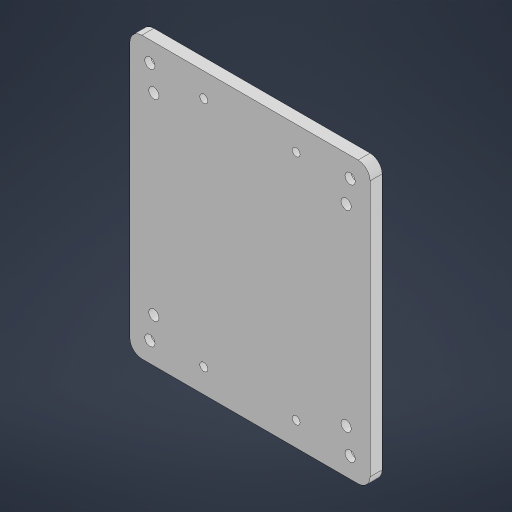
# Autodesk Inventor part: ThirdPlate
Saved by Autodesk Inventor 2024.2 (Build 282272000, 272)
## iProperties
Created: 2023-12-27
Part Number: ThirdPlate
Material: 一般
Document SubType Name: Modeling
Designer: Hanaoka
Density: 1 g/cm^3
Appearance: 既定
Author: Hanaoka
Autodesk Inventor part; units mm, degrees
ref_plane "YZ Plane" through (0, 0, 0) normal (1, 0, 0) x (0, 1, 0)
ref_plane "XZ Plane" through (0, 0, 0) normal (0, 1, 0) x (-1, 0, 0)
ref_plane "XY Plane" through (0, 0, 0) normal (0, 0, 1) x (1, 0, 0)
sketch "スケッチ4" plane through (0, 0, 0) normal (0, 0, 1) x (1, 0, 0)
  line L0 (-27, -35) -> (27, -35)
  line L1 (30, -32) -> (30, 32)
  line L2 (27, 35) -> (-27, 35)
  line L3 (-30, 32) -> (-30, -32)
  line L4 (-30, -35) -> (30, 35) construction
  line L5 (30, -35) -> (-30, 35) construction
  line L6 (-25, -30) -> (25, -30) construction
  line L7 (25, -30) -> (25, 30) construction
  line L8 (25, 30) -> (-25, 30) construction
  line L9 (-25, 30) -> (-25, -30) construction
  line L10 (-25, -30) -> (25, 30) construction
  line L11 (25, -30) -> (-25, 30) construction
  circle A0 centre (-25, 30) radius 1.3
  circle A1 centre (25, 30) radius 1.3
  circle A2 centre (25, -30) radius 1.3
  circle A3 centre (-25, -30) radius 1.3
  circle A4 centre (-25, 30) radius 2.6
  circle A5 centre (25, 30) radius 2.6
  circle A6 centre (25, -30) radius 2.6
  circle A7 centre (-25, -30) radius 2.6
  arc A8 (27, -35) -> (30, -32) centre (27, -32) ccw
  arc A9 (-30, -32) -> (-27, -35) centre (-27, -32) ccw
  arc A10 (-27, 35) -> (-30, 32) centre (-27, 32) ccw
  arc A11 (30, 32) -> (27, 35) centre (27, 32) ccw
  line L12 (24, 24) -> (-24, 24) construction
  line L13 (-24, 24) -> (-24, -24) construction
  line L14 (-24, -24) -> (24, -24) construction
  line L15 (24, -24) -> (24, 24) construction
  line L16 (24, 24) -> (-24, -24) construction
  line L17 (-24, 24) -> (24, -24) construction
  circle A12 centre (-24, -24) radius 1.3
  circle A13 centre (-24, 24) radius 1.3
  circle A14 centre (24, -24) radius 1.3
  circle A15 centre (24, 24) radius 1.3
  point P0 (0, 0)
  dimension "d18" = 70
  dimension "d19" = 60
  dimension "d20" = 50
  dimension "d21" = 60
  dimension "d22" = 2.6
  dimension "d30" = 5.2
  dimension "d33" = 3
  dimension "d40" = 48
  dimension "d41" = 48
  dimension "d42" = 2.6
  constraints: 36 end point, 16 centre point, 12 equal radius, 11 coincident, 8 point on circle, 8 point on line, 8 tangent, 6 midpoint, 6 parallel, 3 horizontal, 3 perpendicular
  measures "d18" distance of L5.start L4.end
  measures "d19" distance of L4.end L5.end
  measures "d20" distance of L7.end L8.end
  measures "d21" distance of L6.end L7.end
  measures "d22" diameter of A0
  measures "d30" diameter of A5
  measures "d33" radius of A8
  measures "d40" distance of L12.end L13.end
  measures "d41" distance of L13.end L14.end
  measures "d42" diameter of A12
extrude "押し出し4" add sketch "スケッチ4" along normal blind 3 contours A9 L3 A10 L2 A11 L1 A8 L0 | A4 | A5 | A6 | A7
extrude "押し出し6" cut sketch "スケッチ4" along normal blind 1.5 contours A0 | A1 | A2 | A3 | A4 | A5 | A6 | A7 | A12 | A13
sketch "スケッチ7" plane through (0, 0, 3) normal (0, 0, 1) x (1, 0, 0)
  line L0 (11.525, -29) -> (-11.525, -29) construction
  line L1 (-11.525, -29) -> (-11.525, 29) construction
  line L2 (-11.525, 29) -> (11.525, 29) construction
  line L3 (11.525, 29) -> (11.525, -29) construction
  line L4 (11.525, -29) -> (-11.525, 29) construction
  line L5 (-11.525, -29) -> (11.525, 29) construction
  circle A0 centre (-11.525, -29) radius 1
  circle A1 centre (-11.525, 29) radius 1
  circle A2 centre (11.525, 29) radius 1
  circle A3 centre (11.525, -29) radius 1
  point P0 (0, 0)
  dimension "d43" = 58
  dimension "d44" = 23.05
  dimension "d45" = 2
  constraints: 12 end point, 4 centre point, 4 coincident, 3 equal radius, 2 midpoint, 2 parallel, 1 horizontal, 1 perpendicular
  measures "d43" distance of L0.end L1.end
  measures "d44" distance of L1.end L2.end
  measures "d45" diameter of A3
extrude "押し出し8" cut sketch "スケッチ7" against normal up to surface (3 mm away)
